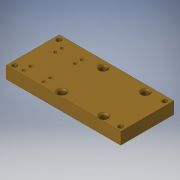
# Autodesk Inventor part: OneSparkMaxPlate
Saved by Autodesk Inventor 2019 (Build 230136000, 136)
## iProperties
Created: 2017-09-23
Part Number: OneSparkMaxPlate
Material: Generic
Document SubType Name: Modeling
Designer: james
Density: 1 g/cm^3
Appearance: Brass - Satin
Author: james
Autodesk Inventor part; units mm, degrees
ref_plane "YZ Plane" through (0, 0, 0) normal (1, 0, 0) x (0, 1, 0)
ref_plane "XZ Plane" through (0, 0, 0) normal (0, 1, 0) x (-1, 0, 0)
ref_plane "XY Plane" through (0, 0, 0) normal (0, 0, 1) x (1, 0, 0)
sketch "Sketch1" plane through (0, 0, 0) normal (0, 1, 0) x (-1, 0, 0)
  line L0 (46.6228, 34.6302) -> (-74.0272, 34.6302)
  line L1 (-74.0272, 34.6302) -> (-74.0272, -54.2698)
  line L2 (-74.0272, -54.2698) -> (46.6228, -54.2698)
  line L3 (46.6228, -54.2698) -> (46.6228, 34.6302)
  point P0 (0, 0)
  dimension "d0" = 120.65
  dimension "d1" = 88.9
  constraints: 8 end point, 2 parallel, 1 horizontal, 1 perpendicular
  measures "d0" distance of L0.start L0.end
  measures "d1" distance of L2.end L0.start
extrude "Extrusion1" add sketch "Sketch1" along normal blind 12.7
sketch "Sketch2" plane through (0, 12.7, 0) normal (0, 1, 0) x (1, 0, 0)
  line L0 (-46.6228, -34.6302) -> (74.0272, -34.6302) projected
  line L1 (-46.6228, 54.2698) -> (-46.6228, -34.6302) projected
  point P0 (0, 0)
  point P1 (6.7172, -29.5502)
  point P2 (51.1672, -29.5502)
  dimension "d4" = 0
  dimension "d5" = 5.08
  dimension "d6" = 53.34
  dimension "d7" = 44.45
  measures "d4" vertical distance of point (51.167, -29.55) point (6.717, -29.55)
  measures "d5" distance from line of L0 point (6.717, -29.55)
  measures "d6" distance from line of L1 point (6.717, -29.55)
  measures "d7" distance of point (51.167, -29.55) point (6.717, -29.55)
hole "Hole1" at (6.7172, 12.7, 29.5502) at (51.1672, 12.7, 29.5502) direction (0, -1, 0) diameter 4.826 depth 25.4 tip angle 118 countersink diameter 9.525 countersink angle 82
sketch "Sketch6" plane through (0, 0, 0) normal (0, -1, 0) x (1, 0, 0)
  line L0 (-46.6228, 34.6302) -> (74.0272, 34.6302) projected
  line L1 (-46.6228, -54.2698) -> (-46.6228, 34.6302) projected
  line L2 (74.0272, -54.2698) -> (-46.6228, -54.2698) projected
  point P0 (0, 0)
  point P1 (69.7092, -16.1698)
  point P2 (-42.0508, -16.1698)
  point P3 (-42.0508, 30.4392)
  point P4 (69.7092, 30.4392)
  dimension "d43" = 0
  dimension "d44" = 0
  dimension "d46" = 111.76
  dimension "d47" = 0
  dimension "d48" = 0
  dimension "d50" = 4.191
  dimension "d51" = 4.572
  dimension "d91" = 38.1
  measures "d43" horizontal distance of point (69.709, -16.17) point (69.709, 30.439)
  measures "d44" vertical distance of point (-42.051, 30.439) point (69.709, 30.439)
  measures "d46" distance of point (69.709, 30.439) point (-42.051, 30.439)
  measures "d47" horizontal distance of point (-42.051, 30.439) point (-42.051, -16.17)
  measures "d48" vertical distance of point (69.709, -16.17) point (-42.051, -16.17)
  measures "d50" distance from line of L0 point (-42.051, 30.439)
  measures "d51" distance from line of L1 point (-42.051, 30.439)
  measures "d91" distance from line of L2 point (-42.051, -16.17)
hole "Hole4" at (69.7092, 0, -16.1698) at (-42.0508, 0, -16.1698) at (-42.0508, 0, 30.4392) at (69.7092, 0, 30.4392) direction (0, 1, 0) diameter 4.8 depth 25.4 tip angle 118
sketch "Sketch10" plane through (0, 12.7, 0) normal (0, 1, 0) x (1, 0, 0)
  circle A0 centre (51.1672, -29.5502) radius 2.413 projected
  circle A1 centre (6.7172, -29.5502) radius 2.413 projected
  line L0 (74.0272, 54.2698) -> (-46.6228, 54.2698) projected
  point P0 (0, 0)
  point P1 (6.7172, 14.2648)
  point P2 (51.1672, 14.2648)
  point P3 (66.6772, 28.8698)
  point P4 (-45.6228, 28.8698)
  point P5 (-46.6228, 54.2698)
  dimension "d80" = 0
  dimension "d81" = 0
  dimension "d82" = 0
  dimension "d144" = 43.815
  constraints: 1 other
  measures "d80" horizontal distance of A1.centre point (6.717, 14.265)
  measures "d81" horizontal distance of point (51.167, 14.265) A0.centre
  measures "d82" vertical distance of point (6.717, 14.265) point (51.167, 14.265)
  measures "d144" distance of point (6.717, 14.265) A1.centre
hole "Hole7" at (6.7172, 12.7, -14.2648) at (51.1672, 12.7, -14.2648) direction (0, -1, 0) diameter 4.826 end through all countersink diameter 9.525 countersink angle 82
sketch "Sketch11" plane through (0, 0, 0) normal (0, -1, 0) x (1, 0, 0)
  line L0 (-28.8428, 29.2002) -> (-16.8428, 29.2002)
  line L1 (-16.8428, 29.2002) -> (-16.8428, 23.2002)
  line L2 (-16.8428, 23.2002) -> (-28.8428, 23.2002)
  line L3 (-28.8428, 23.2002) -> (-28.8428, 29.2002)
  line L4 (-28.8428, -3.8198) -> (-16.8428, -3.8198)
  line L5 (-16.8428, -3.8198) -> (-16.8428, -9.8198)
  line L6 (-16.8428, -9.8198) -> (-28.8428, -9.8198)
  line L7 (-28.8428, -9.8198) -> (-28.8428, -3.8198)
  line L8 (-28.8428, 23.5502) -> (-28.8428, 29.5502) projected
  line L9 (-16.8428, 29.5502) -> (-16.8428, 23.5502) projected
  line L10 (74.0272, -54.2698) -> (-46.6228, -54.2698) projected
  point P0 (0, 0)
  dimension "d93" = 0
  dimension "d94" = 0
  dimension "d95" = 0
  dimension "d96" = 0
  dimension "d97" = 6
  dimension "d98" = 6
  dimension "d99" = 44.45
  dimension "d100" = 77.47
  constraints: 16 end point, 4 parallel, 2 horizontal, 2 perpendicular
  measures "d93" distance between parallel lines of L3 L8
  measures "d94" distance between parallel lines of L9 L1
  measures "d95" distance between parallel lines of L1 L5
  measures "d96" distance between parallel lines of L3 L7
  measures "d97" distance of L2.end L0.start
  measures "d98" distance of L6.end L4.start
  measures "d99" distance between parallel lines of L10 L6
  measures "d100" distance between parallel lines of L2 L10
extrude "Extrusion4" cut sketch "Sketch11" against normal blind 1.27
sketch "Sketch12" plane through (0, 0, 0) normal (0, -1, 0) x (1, 0, 0)
  circle A0 centre (-42.0508, 30.4392) radius 2.4 projected
  circle A1 centre (69.7092, 30.4392) radius 2.4 projected
  circle A2 centre (69.7092, -16.1698) radius 2.4 projected
  circle A3 centre (-42.0508, -16.1698) radius 2.4 projected
  point P0 (0, 0)
  constraints: 4 coincident
hole "Hole8" at (-42.0508, 0, 30.4392) at (69.7092, 0, 30.4392) at (69.7092, 0, -16.1698) at (-42.0508, 0, -16.1698) direction (0, 1, 0) diameter 4.826 end through all
sketch "Sketch13" plane through (0, 0, 0) normal (0, -1, 0) x (1, 0, 0)
  circle A0 centre (-32.8428, -42.0898) radius 1.4 projected
  circle A1 centre (-32.8428, -49.1898) radius 1.4 projected
  line L0 (-46.6228, 34.6302) -> (74.0272, 34.6302) projected
  circle A2 centre (-11.9428, -42.0898) radius 1.4 projected
  point P0 (0, 0)
  point P1 (-32.8428, -10.3398)
  point P2 (-32.8428, -3.2278)
  point P3 (-32.8428, 22.9462)
  point P4 (-32.8428, 30.0582)
  point P5 (-39.7887, 34.6302)
  point P6 (67.4471, 34.6302)
  point P7 (-11.9428, -10.3398)
  point P8 (-11.9428, -3.2278)
  point P9 (-11.9428, 22.9462)
  point P10 (-11.9428, 30.0582)
  dimension "d110" = 0
  dimension "d111" = 0
  dimension "d112" = 0
  dimension "d113" = 7.112
  dimension "d114" = 7.112
  dimension "d115" = 31.75
  dimension "d116" = 4.572
  dimension "d117" = 0
  dimension "d118" = 0
  dimension "d119" = 0
  dimension "d120" = 0
  dimension "d121" = 0
  dimension "d122" = 0
  dimension "d123" = 0
  dimension "d124" = 0
  measures "d110" horizontal distance of point (-32.843, 22.946) point (-32.843, 30.058)
  measures "d111" horizontal distance of point (-32.843, 22.946) point (-32.843, -3.228)
  measures "d112" horizontal distance of point (-32.843, -3.228) point (-32.843, -10.34)
  measures "d113" distance of point (-32.843, -3.228) point (-32.843, -10.34)
  measures "d114" distance of point (-32.843, 30.058) point (-32.843, 22.946)
  measures "d115" distance of point (-32.843, -10.34) A0.centre
  measures "d116" distance from line of point (-32.843, 30.058) L0
  measures "d117" horizontal distance of point (-11.943, -3.228) point (-11.943, -10.34)
  measures "d118" horizontal distance of point (-11.943, 22.946) point (-11.943, -3.228)
  measures "d119" horizontal distance of point (-11.943, 30.058) point (-11.943, 22.946)
  measures "d120" horizontal distance of A2.centre point (-11.943, -10.34)
  measures "d121" vertical distance of point (-11.943, 30.058) point (-32.843, 30.058)
  measures "d122" vertical distance of point (-32.843, 22.946) point (-11.943, 22.946)
  measures "d123" vertical distance of point (-32.843, -3.228) point (-11.943, -3.228)
  measures "d124" vertical distance of point (-32.843, -10.34) point (-11.943, -10.34)
hole "Hole9" at (-32.8428, 0, -10.3398) at (-32.8428, 0, -3.2278) at (-32.8428, 0, 22.9462) at (-32.8428, 0, 30.0582) at (-11.9428, 0, -10.3398) at (-11.9428, 0, -3.2278) at (-11.9428, 0, 22.9462) at (-11.9428, 0, 30.0582) direction (0, 1, 0) diameter 2.8 end through all
sketch "Sketch15" plane through (0, 12.7, 0) normal (0, 1, 0) x (1, 0, 0)
  circle A0 centre (6.7172, 14.2648) radius 2.413 projected
  circle A1 centre (51.1672, 14.2648) radius 2.413 projected
  circle A2 centre (6.7172, -29.5502) radius 2.413 projected
  circle A3 centre (51.1672, -29.5502) radius 2.413 projected
  circle A4 centre (6.7172, 14.2648) radius 3.3734
  circle A5 centre (6.7172, -29.5502) radius 3.3734
  circle A6 centre (51.1672, -29.5502) radius 3.3734
  circle A7 centre (51.1672, 14.2648) radius 3.3734
  point P0 (0, 0)
  dimension "d138" = 6.7469
  dimension "d139" = 6.7469
  dimension "d140" = 6.7469
  dimension "d141" = 6.7469
  constraints: 4 centre point, 4 coincident
  measures "d138" diameter of A4
  measures "d139" diameter of A7
  measures "d140" diameter of A6
  measures "d141" diameter of A5
extrude "Extrusion6" cut sketch "Sketch15" against normal blind 8.89
sketch "Sketch16" plane through (0, 0, 0) normal (0, -1, 0) x (1, 0, 0)
  line L0 (-64.483, -21.2498) -> (91.0848, -21.2498)
  line L1 (91.0848, -21.2498) -> (91.0848, -72.9236)
  line L2 (91.0848, -72.9236) -> (-64.483, -72.9236)
  line L3 (-64.483, -72.9236) -> (-64.483, -21.2498)
  line L4 (74.0272, -54.2698) -> (-46.6228, -54.2698) projected
  point P0 (0, 0)
  dimension "d145" = 33.02
  constraints: 8 end point, 2 parallel, 1 horizontal, 1 perpendicular
  measures "d145" distance between parallel lines of L0 L4
extrude "Extrusion7" cut sketch "Sketch16" against normal blind 25.4
equation "\"d52\" = LegoMainHole"
equation "\"d125\" = CanConHoleDiam"
equation "\"LegoMainHole\" = 4.8"
equation "\"TalonSRXWidth\" = 31.75"
equation "\"TalonSRXFromSide\" = 15.875"
equation "\"TalonSRXBetweenHoles\" = 50.8"
equation "\"CanConPinWidth\" = 6"
equation "\"CanConPinLength\" = 12"
equation "\"CanConBetweenSideHoles\" = 20.9"
equation "\"CanConBetweenTopHoles\" = 7.1"
equation "\"CanConHoleDiam\" = 2.8"
equation "\"CanConHoleFromTopPin\" = 4"
body "Solid1"
